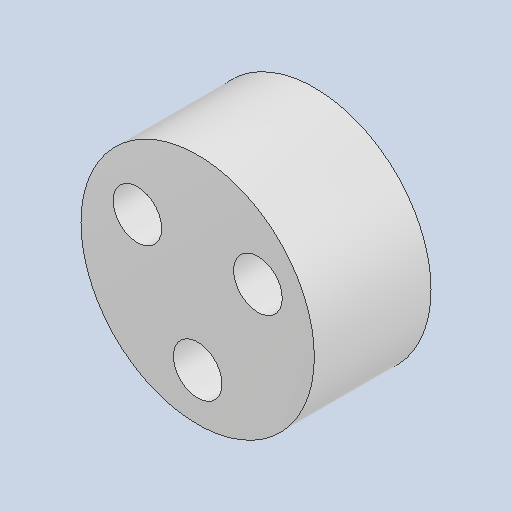
# Autodesk Inventor part: カム
Saved by Autodesk Inventor 2023 (Build 270158000, 158)
## iProperties
Created: 2021-09-13
Part Number: カム
Material: Aluminum 2014-T6
Document SubType Name: Modeling
Designer: muzho
Density: 2.78927 g/cm^3
Appearance: Satin
Author: muzho
Autodesk Inventor part; units mm, degrees
ref_plane "YZ Plane" through (0, 0, 0) normal (1, 0, 0) x (0, 1, 0)
ref_plane "XZ Plane" through (0, 0, 0) normal (0, 1, 0) x (-1, 0, 0)
ref_plane "XY Plane" through (0, 0, 0) normal (0, 0, 1) x (1, 0, 0)
sketch "Sketch1" plane through (0, 0, 0) normal (0, 0, 1) x (1, 0, 0)
  circle A0 centre (-11.7492, -13.0595) radius 1.25
  circle A1 centre (-17.9492, -13.0595) radius 1.25
  circle A2 centre (-14.8492, -18.4288) radius 1.25
  circle A3 centre (-14.8492, -14.8492) radius 6
  point P0 (0, 0)
  point P1 (0, 0)
  dimension "d0" = 12
  constraints: 4 centre point, 1 coincident, 7 other
  measures "d0" diameter of A3
extrude "Extrusion1" add sketch "Sketch1" along normal blind 6
body "Solid1"
